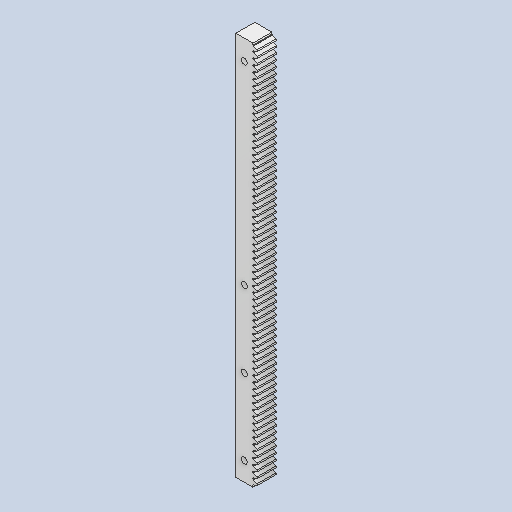
# Autodesk Inventor part: ラックM1‗8
Saved by Autodesk Inventor 2023 (Build 270158000, 158)
## iProperties
Created: 2022-09-12
Part Number: ラックM1‗8
Material: PC/ABS プラスチック
Document SubType Name: Modeling
Designer: 野口　裕太
Density: 0.357273 g/cm^3
Appearance: 滑らか - 白
Author: 野口　裕太
Autodesk Inventor part; units mm, degrees
(part 1 of 4)
ref_plane "YZ Plane" through (0, 0, 0) normal (1, 0, 0) x (0, 1, 0)
ref_plane "XZ Plane" through (0, 0, 0) normal (0, 1, 0) x (-1, 0, 0)
ref_plane "XY Plane" through (0, 0, 0) normal (0, 0, 1) x (1, 0, 0)
sketch "スケッチ1" plane through (0, 0, 0) normal (0, 0, 1) x (1, 0, 0)
  line L0 (8.75, 0) -> (8.75, 0.1735)
  line L1 (8.75, 0.1735) -> (8.7511, 0.1906)
  line L2 (8.7511, 0.1906) -> (8.7542, 0.2077)
  line L3 (8.7542, 0.2077) -> (8.7595, 0.2248)
  line L4 (8.7595, 0.2248) -> (8.7669, 0.2417)
  line L5 (8.7669, 0.2417) -> (8.7764, 0.2586)
  line L6 (8.7764, 0.2586) -> (8.788, 0.2753)
  line L7 (8.788, 0.2753) -> (8.8018, 0.2918)
  line L8 (8.8018, 0.2918) -> (8.8176, 0.3081)
  line L9 (8.8176, 0.3081) -> (8.8355, 0.3242)
  line L10 (8.8355, 0.3242) -> (8.8556, 0.34)
  line L11 (8.8556, 0.34) -> (8.8777, 0.3556)
  line L12 (8.8777, 0.3556) -> (8.9019, 0.3708)
  line L13 (8.9019, 0.3708) -> (8.9282, 0.3857)
  line L14 (8.9282, 0.3857) -> (8.9566, 0.4002)
  line L15 (8.9566, 0.4002) -> (8.9871, 0.4143)
  line L16 (8.9871, 0.4143) -> (9.0196, 0.428)
  line L17 (9.0196, 0.428) -> (9.0542, 0.4412)
  line L18 (9.0542, 0.4412) -> (11, 1.1494)
  line L19 (11, 1.1494) -> (11, 1.5708)
  line L20 (8.788, 2.8663) -> (8.8018, 2.8498)
  line L21 (8.8018, 2.8498) -> (8.8176, 2.8335)
  line L22 (8.8176, 2.8335) -> (8.8355, 2.8174)
  line L23 (8.8355, 2.8174) -> (8.8556, 2.8016)
  line L24 (8.8556, 2.8016) -> (8.8777, 2.786)
  line L25 (8.9019, 2.7708) -> (8.9282, 2.7559)
  line L26 (8.9282, 2.7559) -> (8.9566, 2.7414)
  line L27 (8.9566, 2.7414) -> (8.9871, 2.7273)
  line L28 (8.9871, 2.7273) -> (9.0196, 2.7136)
  line L29 (9.0196, 2.7136) -> (9.0542, 2.7004)
  line L30 (9.0542, 2.7004) -> (11, 1.9922)
  line L31 (11, 1.9922) -> (11, 1.5708)
  line L32 (8.75, 3.1416) -> (8.75, 2.9681)
  line L33 (8.75, 2.9681) -> (8.7511, 2.951)
  line L34 (8.7511, 2.951) -> (8.7542, 2.9339)
  line L35 (8.7764, 2.883) -> (8.788, 2.8663)
  line L36 (8.7669, 2.8999) -> (8.7764, 2.883)
  line L37 (8.7595, 2.9168) -> (8.7669, 2.8999)
  line L38 (8.7542, 2.9339) -> (8.7595, 2.9168)
  line L39 (8.8777, 2.786) -> (8.9019, 2.7708)
  line L40 (8.75, 3.1416) -> (7.1265, 3.1416)
  line L41 (8.8777, 5.9276) -> (8.9019, 5.9124)
  line L42 (8.9019, 5.9124) -> (8.9282, 5.8975)
  line L43 (8.9282, 5.8975) -> (8.9566, 5.883)
  line L44 (8.9566, 5.883) -> (8.9871, 5.8689)
  line L45 (8.9871, 5.8689) -> (9.0196, 5.8552)
  line L46 (9.0196, 5.8552) -> (9.0542, 5.842)
  line L47 (9.0542, 5.842) -> (11, 5.1338)
  line L48 (11, 5.1338) -> (11, 4.7124)
  line L49 (9.0542, 3.5828) -> (11, 4.291)
  line L50 (8.75, 6.2832) -> (8.75, 6.1097)
  line L51 (8.75, 6.1097) -> (8.7511, 6.0926)
  line L52 (8.7511, 6.0926) -> (8.7542, 6.0755)
  line L53 (8.7542, 6.0755) -> (8.7595, 6.0584)
  line L54 (8.8556, 5.9431) -> (8.8777, 5.9276)
  line L55 (8.8355, 5.959) -> (8.8556, 5.9431)
  line L56 (8.8176, 5.9751) -> (8.8355, 5.959)
  line L57 (8.8018, 5.9914) -> (8.8176, 5.9751)
  line L58 (8.788, 6.0079) -> (8.8018, 5.9914)
  line L59 (8.7764, 6.0246) -> (8.788, 6.0079)
  line L60 (8.7669, 6.0415) -> (8.7764, 6.0246)
  line L61 (8.7595, 6.0584) -> (8.7669, 6.0415)
  line L62 (8.9871, 3.5559) -> (9.0196, 3.5695)
  line L63 (8.9566, 3.5418) -> (8.9871, 3.5559)
  line L64 (8.9282, 3.5273) -> (8.9566, 3.5418)
  line L65 (8.9019, 3.5124) -> (8.9282, 3.5273)
  line L66 (8.8777, 3.4972) -> (8.9019, 3.5124)
  line L67 (8.8556, 3.4816) -> (8.8777, 3.4972)
  line L68 (8.8355, 3.4658) -> (8.8556, 3.4816)
  line L69 (8.8176, 3.4497) -> (8.8355, 3.4658)
  line L70 (8.8018, 3.4334) -> (8.8176, 3.4497)
  line L71 (11, 4.291) -> (11, 4.7124)
  line L72 (9.0196, 3.5695) -> (9.0542, 3.5828)
  line L73 (8.788, 3.4169) -> (8.8018, 3.4334)
  line L74 (8.7764, 3.4002) -> (8.788, 3.4169)
  line L75 (8.7595, 3.3664) -> (8.7669, 3.3833)
  line L76 (8.7542, 3.3493) -> (8.7595, 3.3664)
  line L77 (8.7511, 3.3322) -> (8.7542, 3.3493)
  line L78 (8.75, 3.3151) -> (8.7511, 3.3322)
  line L79 (8.75, 3.1416) -> (8.75, 3.3151)
  line L80 (8.7669, 3.3833) -> (8.7764, 3.4002)
  line L81 (8.75, 6.2832) -> (7.8414, 6.2832)
  line L82 (8.9282, 12.1807) -> (8.9566, 12.1662)
  line L83 (8.9566, 12.1662) -> (8.9871, 12.1521)
  line L84 (8.9871, 12.1521) -> (9.0196, 12.1384)
  line L85 (9.0196, 12.1384) -> (9.0542, 12.1252)
  line L86 (9.0542, 12.1252) -> (11, 11.417)
  line L87 (11, 11.417) -> (11, 10.9956)
  line L88 (11, 10.5741) -> (11, 10.9956)
  line L89 (9.0542, 9.8659) -> (11, 10.5741)
  line L90 (9.0196, 9.8527) -> (9.0542, 9.8659)
  line L91 (8.9871, 9.8391) -> (9.0196, 9.8527)
  line L92 (8.9566, 9.825) -> (8.9871, 9.8391)
  line L93 (8.9282, 9.8105) -> (8.9566, 9.825)
  line L94 (8.9019, 9.7956) -> (8.9282, 9.8105)
  line L95 (8.8777, 9.7804) -> (8.9019, 9.7956)
  line L96 (8.788, 9.7001) -> (8.8018, 9.7166)
  line L97 (8.8018, 9.7166) -> (8.8176, 9.7329)
  line L98 (8.8556, 9.7648) -> (8.8777, 9.7804)
  line L99 (8.8355, 9.749) -> (8.8556, 9.7648)
  line L100 (8.8176, 9.7329) -> (8.8355, 9.749)
  line L101 (8.7764, 9.6834) -> (8.788, 9.7001)
  line L102 (8.7669, 9.6665) -> (8.7764, 9.6834)
  line L103 (8.7595, 9.6495) -> (8.7669, 9.6665)
  line L104 (8.7542, 9.6325) -> (8.7595, 9.6495)
  line L105 (8.7511, 9.6154) -> (8.7542, 9.6325)
  line L106 (8.75, 9.5983) -> (8.7511, 9.6154)
  line L107 (8.75, 9.4248) -> (8.75, 9.5983)
  line L108 (8.75, 9.4248) -> (8.75, 9.2513)
  line L109 (8.75, 9.2513) -> (8.7511, 9.2342)
  line L110 (8.7511, 9.2342) -> (8.7542, 9.2171)
  line L111 (8.7542, 9.2171) -> (8.7595, 9.2)
  line L112 (8.7595, 9.2) -> (8.7669, 9.183)
  line L113 (8.7669, 9.183) -> (8.7764, 9.1662)
  line L114 (8.7764, 9.1662) -> (8.788, 9.1495)
  line L115 (8.8018, 9.133) -> (8.8176, 9.1167)
  line L116 (8.8176, 9.1167) -> (8.8355, 9.1006)
  line L117 (8.8355, 9.1006) -> (8.8556, 9.0847)
  line L118 (8.8556, 9.0847) -> (8.8777, 9.0692)
  line L119 (8.8777, 9.0692) -> (8.9019, 9.054)
  line L120 (8.9019, 9.054) -> (8.9282, 9.0391)
  line L121 (8.788, 9.1495) -> (8.8018, 9.133)
  line L122 (8.75, 12.5664) -> (8.75, 12.3929)
  line L123 (8.75, 12.3929) -> (8.7511, 12.3758)
  line L124 (8.7511, 12.3758) -> (8.7542, 12.3586)
  line L125 (8.7542, 12.3586) -> (8.7595, 12.3416)
  line L126 (8.9019, 12.1956) -> (8.9282, 12.1807)
  line L127 (8.8777, 12.2108) -> (8.9019, 12.1956)
  line L128 (8.8556, 12.2263) -> (8.8777, 12.2108)
  line L129 (8.8355, 12.2422) -> (8.8556, 12.2263)
  line L130 (8.8176, 12.2583) -> (8.8355, 12.2422)
  line L131 (8.8018, 12.2746) -> (8.8176, 12.2583)
  line L132 (8.788, 12.2911) -> (8.8018, 12.2746)
  line L133 (8.7764, 12.3078) -> (8.788, 12.2911)
  line L134 (8.7669, 12.3246) -> (8.7764, 12.3078)
  line L135 (8.7595, 12.3416) -> (8.7669, 12.3246)
  line L136 (8.8777, 6.6388) -> (8.9019, 6.654)
  line L137 (8.9019, 6.654) -> (8.9282, 6.6689)
  line L138 (8.75, 6.2832) -> (8.75, 6.4567)
  line L139 (8.75, 6.4567) -> (8.7511, 6.4738)
  line L140 (8.7511, 6.4738) -> (8.7542, 6.4909)
  line L141 (8.7542, 6.4909) -> (8.7595, 6.508)
  line L142 (8.8556, 6.6232) -> (8.8777, 6.6388)
  line L143 (8.8355, 6.6074) -> (8.8556, 6.6232)
  line L144 (8.8176, 6.5913) -> (8.8355, 6.6074)
  line L145 (8.8018, 6.575) -> (8.8176, 6.5913)
  line L146 (8.788, 6.5585) -> (8.8018, 6.575)
  line L147 (8.7764, 6.5418) -> (8.788, 6.5585)
  line L148 (8.7669, 6.5249) -> (8.7764, 6.5418)
  line L149 (8.7595, 6.508) -> (8.7669, 6.5249)
  line L150 (8.9282, 6.6689) -> (8.9566, 6.6834)
  line L151 (8.9566, 6.6834) -> (8.9871, 6.6975)
  line L152 (8.9871, 6.6975) -> (9.0196, 6.7111)
  line L153 (9.0196, 6.7111) -> (9.0542, 6.7243)
  line L154 (9.0542, 6.7243) -> (11, 7.4326)
  line L155 (11, 7.4326) -> (11, 7.854)
  line L156 (9.0542, 8.9836) -> (11, 8.2754)
  line L157 (8.9871, 9.0105) -> (9.0196, 8.9968)
  line L158 (8.9566, 9.0246) -> (8.9871, 9.0105)
  line L159 (9.0196, 8.9968) -> (9.0542, 8.9836)
  line L160 (11, 8.2754) -> (11, 7.854)
  line L161 (8.9282, 9.0391) -> (8.9566, 9.0246)
  line L162 (8.75, 12.5664) -> (7.1265, 12.5664)
  line L163 (8.9871, 24.7185) -> (9.0196, 24.7048)
  line L164 (9.0196, 24.7048) -> (9.0542, 24.6916)
  line L165 (9.0542, 24.6916) -> (11, 23.9834)
  line L166 (11, 23.9834) -> (11, 23.5619)
  line L167 (8.75, 25.1327) -> (8.75, 24.9593)
  line L168 (8.75, 24.9593) -> (8.7511, 24.9421)
  line L169 (8.7511, 24.9421) -> (8.7542, 24.925)
  line L170 (8.7542, 24.925) -> (8.7595, 24.908)
  line L171 (8.8176, 24.8246) -> (8.8355, 24.8085)
  line L172 (8.8355, 24.8085) -> (8.8556, 24.7927)
  line L173 (8.9282, 24.7471) -> (8.9566, 24.7326)
  line L174 (8.9019, 24.7619) -> (8.9282, 24.7471)
  line L175 (8.8777, 24.7772) -> (8.9019, 24.7619)
  line L176 (8.8556, 24.7927) -> (8.8777, 24.7772)
  line L177 (8.8018, 24.8409) -> (8.8176, 24.8246)
  line L178 (8.788, 24.8575) -> (8.8018, 24.8409)
  line L179 (8.7764, 24.8742) -> (8.788, 24.8575)
  line L180 (8.7669, 24.891) -> (8.7764, 24.8742)
  line L181 (8.7595, 24.908) -> (8.7669, 24.891)
  line L182 (8.9566, 24.7326) -> (8.9871, 24.7185)
  line L183 (11, 23.1405) -> (11, 23.5619)
  line L184 (9.0542, 22.4323) -> (11, 23.1405)
  line L185 (9.0196, 22.4191) -> (9.0542, 22.4323)
  line L186 (8.9871, 22.4054) -> (9.0196, 22.4191)
  line L187 (8.9566, 22.3913) -> (8.9871, 22.4054)
  line L188 (8.9282, 22.3768) -> (8.9566, 22.3913)
  line L189 (8.9019, 22.362) -> (8.9282, 22.3768)
  line L190 (8.788, 22.2664) -> (8.8018, 22.2829)
  line L191 (8.8018, 22.2829) -> (8.8176, 22.2993)
  line L192 (8.8176, 22.2993) -> (8.8355, 22.3154)
  line L193 (8.8777, 22.3467) -> (8.9019, 22.362)
  line L194 (8.8556, 22.3312) -> (8.8777, 22.3467)
  line L195 (8.8355, 22.3154) -> (8.8556, 22.3312)
  line L196 (8.7764, 22.2497) -> (8.788, 22.2664)
  line L197 (8.7669, 22.2329) -> (8.7764, 22.2497)
  line L198 (8.7595, 22.2159) -> (8.7669, 22.2329)
  line L199 (8.7542, 22.1989) -> (8.7595, 22.2159)
  line L200 (8.7511, 22.1818) -> (8.7542, 22.1989)
  line L201 (8.75, 22.1646) -> (8.7511, 22.1818)
  line L202 (8.75, 21.9911) -> (8.75, 22.1646)
  line L203 (8.7764, 21.7326) -> (8.788, 21.7159)
  line L204 (8.788, 21.7159) -> (8.8018, 21.6994)
  line L205 (8.8018, 21.6994) -> (8.8176, 21.683)
  line L206 (8.8355, 21.6669) -> (8.8556, 21.6511)
  line L207 (8.8556, 21.6511) -> (8.8777, 21.6356)
  line L208 (8.8777, 21.6356) -> (8.9019, 21.6203)
  line L209 (8.9019, 21.6203) -> (8.9282, 21.6055)
  line L210 (8.9282, 21.6055) -> (8.9566, 21.591)
  line L211 (8.8176, 21.683) -> (8.8355, 21.6669)
  line L212 (8.8777, 19.2051) -> (8.9019, 19.2204)
  line L213 (8.9019, 19.2204) -> (8.9282, 19.2352)
  line L214 (8.75, 18.8496) -> (8.75, 19.023)
  line L215 (8.75, 19.023) -> (8.7511, 19.0402)
  line L216 (8.7511, 19.0402) -> (8.7542, 19.0573)
  line L217 (8.7542, 19.0573) -> (8.7595, 19.0743)
  line L218 (8.8556, 19.1896) -> (8.8777, 19.2051)
  line L219 (8.8355, 19.1738) -> (8.8556, 19.1896)
  line L220 (8.8176, 19.1577) -> (8.8355, 19.1738)
  line L221 (8.8018, 19.1414) -> (8.8176, 19.1577)
  line L222 (8.7595, 19.0743) -> (8.7669, 19.0913)
  line L223 (8.7669, 19.0913) -> (8.7764, 19.1081)
  line L224 (8.788, 19.1248) -> (8.8018, 19.1414)
  line L225 (8.7764, 19.1081) -> (8.788, 19.1248)
  line L226 (8.9282, 19.2352) -> (8.9566, 19.2497)
  line L227 (8.9566, 19.2497) -> (8.9871, 19.2638)
  line L228 (8.9871, 19.2638) -> (9.0196, 19.2775)
  line L229 (9.0196, 19.2775) -> (9.0542, 19.2907)
  line L230 (9.0542, 19.2907) -> (11, 19.9989)
  line L231 (11, 19.9989) -> (11, 20.4204)
  line L232 (9.0542, 21.55) -> (11, 20.8418)
  line L233 (8.9871, 21.5769) -> (9.0196, 21.5632)
  line L234 (9.0196, 21.5632) -> (9.0542, 21.55)
  line L235 (11, 20.8418) -> (11, 20.4204)
  line L236 (8.9566, 21.591) -> (8.9871, 21.5769)
  line L237 (8.7669, 21.7494) -> (8.7764, 21.7326)
  line L238 (8.7595, 21.7664) -> (8.7669, 21.7494)
  line L239 (8.7542, 21.7834) -> (8.7595, 21.7664)
  line L240 (8.7511, 21.8005) -> (8.7542, 21.7834)
  line L241 (8.75, 21.8177) -> (8.7511, 21.8005)
  line L242 (8.75, 21.9911) -> (8.75, 21.8177)
  line L243 (8.9566, 12.9666) -> (8.9871, 12.9807)
  line L244 (8.9871, 12.9807) -> (9.0196, 12.9943)
  line L245 (9.0196, 12.9943) -> (9.0542, 13.0075)
  line L246 (9.0542, 15.2668) -> (11, 14.5586)
  line L247 (9.0542, 13.0075) -> (11, 13.7157)
  line L248 (11, 14.5586) -> (11, 14.1372)
  line L249 (11, 13.7157) -> (11, 14.1372)
  line L250 (8.7542, 15.5002) -> (8.7595, 15.4832)
  line L251 (8.7511, 15.5173) -> (8.7542, 15.5002)
  line L252 (8.75, 15.5345) -> (8.7511, 15.5173)
  line L253 (8.75, 15.708) -> (8.75, 15.5345)
  line L254 (8.75, 15.708) -> (8.75, 15.8814)
  line L255 (8.7595, 15.4832) -> (8.7669, 15.4662)
  line L256 (9.0196, 15.28) -> (9.0542, 15.2668)
  line L257 (8.9871, 15.2937) -> (9.0196, 15.28)
  line L258 (8.9566, 15.3078) -> (8.9871, 15.2937)
  line L259 (8.9282, 15.3223) -> (8.9566, 15.3078)
  line L260 (8.9019, 15.3372) -> (8.9282, 15.3223)
  line L261 (8.8777, 15.3524) -> (8.9019, 15.3372)
  line L262 (8.8556, 15.3679) -> (8.8777, 15.3524)
  line L263 (8.8355, 15.3838) -> (8.8556, 15.3679)
  line L264 (8.8176, 15.3998) -> (8.8355, 15.3838)
  line L265 (8.8018, 15.4162) -> (8.8176, 15.3998)
  line L266 (8.788, 15.4327) -> (8.8018, 15.4162)
  line L267 (8.7764, 15.4494) -> (8.788, 15.4327)
  line L268 (8.7669, 15.4662) -> (8.7764, 15.4494)
  line L269 (8.8556, 16.048) -> (8.8777, 16.0635)
  line L270 (8.8777, 16.0635) -> (8.9019, 16.0788)
  line L271 (8.9019, 16.0788) -> (8.9282, 16.0936)
  line L272 (8.9282, 16.0936) -> (8.9566, 16.1082)
  line L273 (8.9566, 16.1082) -> (8.9871, 16.1222)
  line L274 (8.9871, 16.1222) -> (9.0196, 16.1359)
  line L275 (8.75, 15.8814) -> (8.7511, 15.8986)
  line L276 (8.7511, 15.8986) -> (8.7542, 15.9157)
  line L277 (8.7542, 15.9157) -> (8.7595, 15.9327)
  line L278 (8.7595, 15.9327) -> (8.7669, 15.9497)
  line L279 (8.7669, 15.9497) -> (8.7764, 15.9665)
  line L280 (8.7764, 15.9665) -> (8.788, 15.9832)
  line L281 (8.788, 15.9832) -> (8.8018, 15.9998)
  line L282 (8.8018, 15.9998) -> (8.8176, 16.0161)
  line L283 (8.8176, 16.0161) -> (8.8355, 16.0322)
  line L284 (8.8355, 16.0322) -> (8.8556, 16.048)
  line L285 (8.75, 18.8496) -> (8.75, 18.6761)
  line L286 (8.75, 18.6761) -> (8.7511, 18.6589)
  line L287 (8.7511, 18.6589) -> (8.7542, 18.6418)
  line L288 (8.7542, 18.6418) -> (8.7595, 18.6248)
  line L289 (8.7595, 18.6248) -> (8.7669, 18.6078)
  line L290 (8.7764, 18.591) -> (8.788, 18.5743)
  line L291 (8.788, 18.5743) -> (8.8018, 18.5578)
  line L292 (8.8018, 18.5578) -> (8.8176, 18.5414)
  line L293 (8.8176, 18.5414) -> (8.8355, 18.5253)
  line L294 (8.8355, 18.5253) -> (8.8556, 18.5095)
  line L295 (8.8556, 18.5095) -> (8.8777, 18.494)
  line L296 (8.7669, 18.6078) -> (8.7764, 18.591)
  line L297 (8.8777, 18.494) -> (8.9019, 18.4787)
  line L298 (8.9019, 18.4787) -> (8.9282, 18.4639)
  line L299 (8.9282, 18.4639) -> (8.9566, 18.4494)
  line L300 (8.9566, 18.4494) -> (8.9871, 18.4353)
  line L301 (8.9871, 18.4353) -> (9.0196, 18.4216)
  line L302 (9.0196, 18.4216) -> (9.0542, 18.4084)
  line L303 (8.9282, 12.9521) -> (8.9566, 12.9666)
  line L304 (8.9019, 12.9372) -> (8.9282, 12.9521)
  line L305 (8.8777, 12.922) -> (8.9019, 12.9372)
  line L306 (8.8355, 12.8906) -> (8.8556, 12.9064)
  line L307 (8.8176, 12.8745) -> (8.8355, 12.8906)
  line L308 (8.8018, 12.8582) -> (8.8176, 12.8745)
  line L309 (8.788, 12.8416) -> (8.8018, 12.8582)
  line L310 (8.7764, 12.8249) -> (8.788, 12.8416)
  line L311 (8.7669, 12.8081) -> (8.7764, 12.8249)
  line L312 (8.7595, 12.7911) -> (8.7669, 12.8081)
  line L313 (8.7542, 12.7741) -> (8.7595, 12.7911)
  line L314 (8.7511, 12.757) -> (8.7542, 12.7741)
  line L315 (8.75, 12.7399) -> (8.7511, 12.757)
  line L316 (8.75, 12.5664) -> (8.75, 12.7399)
  line L317 (8.8556, 12.9064) -> (8.8777, 12.922)
  line L318 (9.0542, 18.4084) -> (11, 17.7002)
  line L319 (11, 17.7002) -> (11, 17.2788)
  line L320 (9.0196, 16.1359) -> (9.0542, 16.1491)
  line L321 (11, 16.8573) -> (11, 17.2788)
  line L322 (9.0542, 16.1491) -> (11, 16.8573)
  line L323 (8.75, 25.1327) -> (7.9383, 25.1327)
  line L324 (8.75, 50.2655) -> (8.75, 50.092)
  line L325 (8.75, 50.092) -> (8.7511, 50.0749)
  line L326 (8.7511, 50.0749) -> (8.7542, 50.0578)
  line L327 (8.7542, 50.0578) -> (8.7595, 50.0407)
  line L328 (8.7595, 50.0407) -> (8.7669, 50.0238)
  line L329 (8.7669, 50.0238) -> (8.7764, 50.0069)
  line L330 (8.9019, 49.8947) -> (8.9282, 49.8798)
  line L331 (8.9282, 49.8798) -> (8.9566, 49.8653)
  line L332 (8.7764, 50.0069) -> (8.788, 49.9902)
  line L333 (8.9566, 49.8653) -> (8.9871, 49.8512)
  line L334 (8.788, 47.3992) -> (8.8018, 47.4157)
  line L335 (8.8018, 47.4157) -> (8.8176, 47.432)
  line L336 (8.7764, 47.3825) -> (8.788, 47.3992)
  line L337 (8.7669, 47.3656) -> (8.7764, 47.3825)
  line L338 (8.7595, 47.3487) -> (8.7669, 47.3656)
  line L339 (8.7542, 47.3316) -> (8.7595, 47.3487)
  line L340 (8.7511, 47.3145) -> (8.7542, 47.3316)
  line L341 (8.75, 47.2974) -> (8.7511, 47.3145)
  line L342 (8.75, 47.1239) -> (8.75, 47.2974)
  line L343 (8.8176, 47.432) -> (8.8355, 47.4481)
  line L344 (8.9871, 49.8512) -> (9.0196, 49.8375)
  line L345 (9.0196, 49.8375) -> (9.0542, 49.8243)
  line L346 (8.8777, 49.9099) -> (8.9019, 49.8947)
  line L347 (8.8556, 49.9254) -> (8.8777, 49.9099)
  line L348 (8.8355, 49.9413) -> (8.8556, 49.9254)
  line L349 (8.8176, 49.9574) -> (8.8355, 49.9413)
  line L350 (8.8018, 49.9737) -> (8.8176, 49.9574)
  line L351 (9.0542, 49.8243) -> (11, 49.1161)
  line L352 (9.0542, 47.5651) -> (11, 48.2733)
  line L353 (11, 48.2733) -> (11, 48.6947)
  line L354 (11, 49.1161) -> (11, 48.6947)
  line L355 (8.788, 49.9902) -> (8.8018, 49.9737)
  line L356 (8.75, 47.1239) -> (8.75, 46.9504)
  line L357 (8.75, 46.9504) -> (8.7511, 46.9333)
  line L358 (8.7511, 46.9333) -> (8.7542, 46.9162)
  line L359 (8.7542, 46.9162) -> (8.7595, 46.8991)
  line L360 (8.7595, 46.8991) -> (8.7669, 46.8822)
  line L361 (8.7669, 46.8822) -> (8.7764, 46.8653)
  line L362 (8.7764, 46.8653) -> (8.788, 46.8486)
  line L363 (8.788, 46.8486) -> (8.8018, 46.8321)
  line L364 (8.8018, 46.8321) -> (8.8176, 46.8158)
  line L365 (8.8777, 44.3379) -> (8.9019, 44.3531)
  line L366 (8.9019, 44.3531) -> (8.9282, 44.368)
  line L367 (8.9282, 44.368) -> (8.9566, 44.3825)
  line L368 (8.9566, 44.3825) -> (8.9871, 44.3966)
  line L369 (8.7595, 44.2071) -> (8.7669, 44.224)
  line L370 (8.7669, 44.224) -> (8.7764, 44.2409)
  line L371 (8.7764, 44.2409) -> (8.788, 44.2576)
  line L372 (8.788, 44.2576) -> (8.8018, 44.2741)
  line L373 (8.8018, 44.2741) -> (8.8176, 44.2904)
  line L374 (8.8176, 44.2904) -> (8.8355, 44.3065)
  line L375 (8.8556, 44.3223) -> (8.8777, 44.3379)
  line L376 (8.8355, 44.3065) -> (8.8556, 44.3223)
  line L377 (8.9871, 44.3966) -> (9.0196, 44.4103)
  line L378 (9.0196, 44.4103) -> (9.0542, 44.4235)
  line L379 (9.0542, 44.4235) -> (11, 45.1317)
  line L380 (11, 45.1317) -> (11, 45.5531)
  line L381 (9.0542, 46.6827) -> (11, 45.9745)
  line L382 (8.9871, 46.7096) -> (9.0196, 46.6959)
  line L383 (8.8355, 46.7997) -> (8.8556, 46.7838)
  line L384 (8.8556, 46.7838) -> (8.8777, 46.7683)
  line L385 (8.8777, 46.7683) -> (8.9019, 46.7531)
  line L386 (8.9019, 46.7531) -> (8.9282, 46.7382)
  line L387 (8.9282, 46.7382) -> (8.9566, 46.7237)
  line L388 (8.9566, 46.7237) -> (8.9871, 46.7096)
  line L389 (9.0196, 46.6959) -> (9.0542, 46.6827)
  line L390 (11, 45.9745) -> (11, 45.5531)
  line L391 (8.8176, 46.8158) -> (8.8355, 46.7997)
  line L392 (8.8355, 47.4481) -> (8.8556, 47.4639)
  line L393 (8.8556, 47.4639) -> (8.8777, 47.4795)
  line L394 (8.8777, 47.4795) -> (8.9019, 47.4947)
  line L395 (8.9019, 47.4947) -> (8.9282, 47.5096)
  line L396 (8.9282, 47.5096) -> (8.9566, 47.5241)
  line L397 (8.9566, 47.5241) -> (8.9871, 47.5382)
  line L398 (8.9871, 47.5382) -> (9.0196, 47.5518)
  line L399 (9.0196, 47.5518) -> (9.0542, 47.5651)
  line L400 (8.7764, 40.5821) -> (8.788, 40.5654)
  line L401 (8.7669, 40.599) -> (8.7764, 40.5821)
  line L402 (8.7595, 40.6159) -> (8.7669, 40.599)
  line L403 (8.7542, 40.633) -> (8.7595, 40.6159)
  line L404 (8.7511, 40.6501) -> (8.7542, 40.633)
  line L405 (8.75, 40.6672) -> (8.7511, 40.6501)
  line L406 (8.75, 40.8407) -> (8.75, 40.6672)
  line L407 (8.788, 40.5654) -> (8.8018, 40.5489)
  line L408 (8.9871, 38.1134) -> (9.0196, 38.1271)
  line L409 (9.0196, 38.1271) -> (9.0542, 38.1403)
  line L410 (9.0542, 38.1403) -> (11, 38.8485)
  line L411 (11, 38.8485) -> (11, 39.2699)
  line L412 (11, 39.6913) -> (11, 39.2699)
  line L413 (9.0542, 40.3995) -> (11, 39.6913)
  line L414 (9.0196, 40.4128) -> (9.0542, 40.3995)
  line L415 (8.8018, 40.5489) -> (8.8176, 40.5326)
  line L416 (8.8355, 40.5165) -> (8.8556, 40.5007)
  line L417 (8.8556, 40.5007) -> (8.8777, 40.4851)
  line L418 (8.8777, 40.4851) -> (8.9019, 40.4699)
  line L419 (8.9019, 40.4699) -> (8.9282, 40.455)
  line L420 (8.9282, 40.455) -> (8.9566, 40.4405)
  line L421 (8.9566, 40.4405) -> (8.9871, 40.4264)
  line L422 (8.9871, 40.4264) -> (9.0196, 40.4128)
  line L423 (8.8176, 40.5326) -> (8.8355, 40.5165)
  line L424 (8.75, 40.8407) -> (8.75, 41.0142)
  line L425 (8.75, 41.0142) -> (8.7511, 41.0313)
  line L426 (8.7542, 41.0484) -> (8.7595, 41.0655)
  line L427 (8.7595, 41.0655) -> (8.7669, 41.0824)
  line L428 (8.7669, 41.0824) -> (8.7764, 41.0993)
  line L429 (8.7764, 41.0993) -> (8.788, 41.116)
  line L430 (8.7511, 41.0313) -> (8.7542, 41.0484)
  line L431 (8.788, 41.116) -> (8.8018, 41.1325)
  line L432 (8.8176, 41.1488) -> (8.8355, 41.1649)
  line L433 (8.8355, 41.1649) -> (8.8556, 41.1807)
  line L434 (8.8556, 41.1807) -> (8.8777, 41.1963)
  line L435 (8.8777, 41.1963) -> (8.9019, 41.2115)
  line L436 (8.9019, 41.2115) -> (8.9282, 41.2264)
  line L437 (8.9282, 41.2264) -> (8.9566, 41.2409)
  line L438 (8.9566, 41.2409) -> (8.9871, 41.255)
  line L439 (8.8018, 41.1325) -> (8.8176, 41.1488)
  line L440 (8.9282, 38.0848) -> (8.9566, 38.0993)
  line L441 (8.9566, 38.0993) -> (8.9871, 38.1134)
  line L442 (8.75, 37.6991) -> (8.75, 37.8726)
  line L443 (8.75, 37.8726) -> (8.7511, 37.8897)
  line L444 (8.7511, 37.8897) -> (8.7542, 37.9068)
  line L445 (8.7542, 37.9068) -> (8.7595, 37.9239)
  line L446 (8.9019, 38.0699) -> (8.9282, 38.0848)
  line L447 (8.8777, 38.0547) -> (8.9019, 38.0699)
  line L448 (8.8556, 38.0392) -> (8.8777, 38.0547)
  line L449 (8.8355, 38.0233) -> (8.8556, 38.0392)
  line L450 (8.7595, 37.9239) -> (8.7669, 37.9408)
  line L451 (8.7764, 37.9577) -> (8.788, 37.9744)
  line L452 (8.788, 37.9744) -> (8.8018, 37.9909)
  line L453 (8.8018, 37.9909) -> (8.8176, 38.0072)
  line L454 (8.8176, 38.0072) -> (8.8355, 38.0233)
  line L455 (8.7669, 37.9408) -> (8.7764, 37.9577)
  line L456 (8.75, 43.9823) -> (8.75, 44.1558)
  line L457 (8.75, 44.1558) -> (8.7511, 44.1729)
  line L458 (8.7511, 44.1729) -> (8.7542, 44.19)
  line L459 (8.75, 43.9823) -> (8.75, 43.8088)
  line L460 (8.75, 43.8088) -> (8.7511, 43.7917)
  line L461 (8.7511, 43.7917) -> (8.7542, 43.7746)
  line L462 (8.7542, 43.7746) -> (8.7595, 43.7575)
  line L463 (8.7595, 43.7575) -> (8.7669, 43.7406)
  line L464 (8.7669, 43.7406) -> (8.7764, 43.7237)
  line L465 (8.7764, 43.7237) -> (8.788, 43.707)
  line L466 (8.788, 43.707) -> (8.8018, 43.6905)
  line L467 (8.8018, 43.6905) -> (8.8176, 43.6742)
  line L468 (8.7542, 44.19) -> (8.7595, 44.2071)
  line L469 (8.8777, 43.6267) -> (8.9019, 43.6115)
  line L470 (8.8176, 43.6742) -> (8.8355, 43.6581)
  line L471 (8.8355, 43.6581) -> (8.8556, 43.6423)
  line L472 (8.8556, 43.6423) -> (8.8777, 43.6267)
  line L473 (8.9019, 43.6115) -> (8.9282, 43.5966)
  line L474 (8.9282, 43.5966) -> (8.9566, 43.5821)
  line L475 (8.9566, 43.5821) -> (8.9871, 43.568)
  line L476 (8.9871, 43.568) -> (9.0196, 43.5543)
  line L477 (9.0196, 43.5543) -> (9.0542, 43.5411)
  line L478 (9.0196, 41.2687) -> (9.0542, 41.2819)
  line L479 (9.0542, 41.2819) -> (11, 41.9901)
  line L480 (11, 41.9901) -> (11, 42.4115)
  line L481 (11, 42.8329) -> (11, 42.4115)
  line L482 (9.0542, 43.5411) -> (11, 42.8329)
  line L483 (8.9871, 41.255) -> (9.0196, 41.2687)
  line L484 (8.75, 25.3062) -> (8.7511, 25.3234)
  line L485 (8.75, 25.1327) -> (8.75, 25.3062)
  line L486 (9.0542, 25.5739) -> (11, 26.2821)
  line L487 (11, 26.2821) -> (11, 26.7035)
  line L488 (11, 27.125) -> (11, 26.7035)
  line L489 (9.0542, 27.8332) -> (11, 27.125)
  line L490 (9.0196, 27.8464) -> (9.0542, 27.8332)
  line L491 (8.9871, 27.86) -> (9.0196, 27.8464)
  line L492 (8.7764, 28.0158) -> (8.788, 27.9991)
  line L493 (8.788, 27.9991) -> (8.8018, 27.9825)
  line L494 (8.8018, 27.9825) -> (8.8176, 27.9662)
  line L495 (8.8176, 27.9662) -> (8.8355, 27.9501)
  line L496 (8.8355, 27.9501) -> (8.8556, 27.9343)
  line L497 (8.8556, 27.9343) -> (8.8777, 27.9188)
  line L498 (8.8777, 27.9188) -> (8.9019, 27.9035)
  line L499 (8.9019, 27.9035) -> (8.9282, 27.8886)
  line L500 (8.9282, 27.8886) -> (8.9566, 27.8741)
  line L501 (8.9566, 27.8741) -> (8.9871, 27.86)
  line L502 (8.7669, 28.0326) -> (8.7764, 28.0158)
  line L503 (8.7595, 28.0496) -> (8.7669, 28.0326)
  line L504 (8.7542, 28.0666) -> (8.7595, 28.0496)
  line L505 (8.7511, 28.0837) -> (8.7542, 28.0666)
  line L506 (8.75, 28.1008) -> (8.7511, 28.0837)
  line L507 (8.75, 28.2743) -> (8.75, 28.1008)
  line L508 (8.75, 28.2743) -> (8.75, 28.4478)
  line L509 (8.75, 28.4478) -> (8.7511, 28.465)
  line L510 (8.7511, 28.465) -> (8.7542, 28.4821)
  line L511 (8.7542, 28.4821) -> (8.7595, 28.4991)
  line L512 (8.7595, 28.4991) -> (8.7669, 28.5161)
  line L513 (8.7669, 28.5161) -> (8.7764, 28.5329)
  line L514 (8.7764, 28.5329) -> (8.788, 28.5496)
  line L515 (8.788, 28.5496) -> (8.8018, 28.5661)
  line L516 (8.8018, 28.5661) -> (8.8176, 28.5825)
  line L517 (8.8176, 28.5825) -> (8.8355, 28.5985)
  line L518 (8.8355, 28.5985) -> (8.8556, 28.6144)
  line L519 (8.8556, 28.6144) -> (8.8777, 28.6299)
  line L520 (8.9019, 28.6451) -> (8.9282, 28.66)
  line L521 (8.8777, 28.6299) -> (8.9019, 28.6451)
  line L522 (8.8777, 31.0603) -> (8.9019, 31.0451)
  line L523 (8.8176, 31.1078) -> (8.8355, 31.0917)
  line L524 (8.8355, 31.0917) -> (8.8556, 31.0759)
  line L525 (8.8556, 31.0759) -> (8.8777, 31.0603)
  line L526 (8.9019, 31.0451) -> (8.9282, 31.0302)
  line L527 (8.8018, 31.1241) -> (8.8176, 31.1078)
  line L528 (8.788, 31.1407) -> (8.8018, 31.1241)
  line L529 (8.7764, 31.1574) -> (8.788, 31.1407)
  line L530 (8.7669, 31.1742) -> (8.7764, 31.1574)
  line L531 (8.7595, 31.1912) -> (8.7669, 31.1742)
  line L532 (8.7542, 31.2082) -> (8.7595, 31.1912)
  line L533 (8.7511, 31.2253) -> (8.7542, 31.2082)
  line L534 (8.75, 31.2424) -> (8.7511, 31.2253)
  line L535 (8.75, 31.4159) -> (8.75, 31.2424)
  line L536 (8.75, 31.4159) -> (8.75, 31.5894)
  line L537 (8.75, 31.5894) -> (8.7511, 31.6065)
  line L538 (8.7511, 31.6065) -> (8.7542, 31.6236)
  line L539 (8.7542, 31.6236) -> (8.7595, 31.6407)
  line L540 (8.9871, 25.547) -> (9.0196, 25.5607)
  line L541 (9.0196, 25.5607) -> (9.0542, 25.5739)
  line L542 (8.7511, 25.3234) -> (8.7542, 25.3405)
  line L543 (8.7542, 25.3405) -> (8.7595, 25.3575)
  line L544 (8.7595, 25.3575) -> (8.7669, 25.3745)
  line L545 (8.7669, 25.3745) -> (8.7764, 25.3913)
  line L546 (8.7764, 25.3913) -> (8.788, 25.408)
  line L547 (8.788, 25.408) -> (8.8018, 25.4245)
  line L548 (8.8018, 25.4245) -> (8.8176, 25.4409)
  line L549 (8.8176, 25.4409) -> (8.8355, 25.457)
  line L550 (8.8355, 25.457) -> (8.8556, 25.4728)
  line L551 (8.8556, 25.4728) -> (8.8777, 25.4883)
  line L552 (8.9019, 25.5035) -> (8.9282, 25.5184)
  line L553 (8.9282, 25.5184) -> (8.9566, 25.5329)
  line L554 (8.9566, 25.5329) -> (8.9871, 25.547)
  line L555 (8.8777, 25.4883) -> (8.9019, 25.5035)
  line L556 (8.7595, 31.6407) -> (8.7669, 31.6577)
  line L557 (8.7764, 31.6745) -> (8.788, 31.6912)
  line L558 (8.788, 31.6912) -> (8.8018, 31.7077)
  line L559 (8.8018, 31.7077) -> (8.8176, 31.724)
  line L560 (8.8176, 31.724) -> (8.8355, 31.7401)
  line L561 (8.8355, 31.7401) -> (8.8556, 31.756)
  line L562 (8.8556, 31.756) -> (8.8777, 31.7715)
  line L563 (8.7669, 31.6577) -> (8.7764, 31.6745)
  line L564 (8.75, 37.6991) -> (8.75, 37.5256)
  line L565 (8.75, 37.5256) -> (8.7511, 37.5085)
  line L566 (8.7511, 37.5085) -> (8.7542, 37.4914)
  line L567 (8.7542, 37.4914) -> (8.7595, 37.4743)
  line L568 (8.7595, 37.4743) -> (8.7669, 37.4574)
  line L569 (8.7669, 37.4574) -> (8.7764, 37.4405)
  line L570 (8.7764, 37.4405) -> (8.788, 37.4238)
  line L571 (8.788, 37.4238) -> (8.8018, 37.4073)
  line L572 (8.8018, 37.4073) -> (8.8176, 37.391)
  line L573 (8.8176, 37.391) -> (8.8355, 37.3749)
  line L574 (8.8355, 37.3749) -> (8.8556, 37.3591)
  line L575 (8.7511, 34.7481) -> (8.7542, 34.7652)
  line L576 (8.75, 34.731) -> (8.7511, 34.7481)
  line L577 (8.75, 34.5575) -> (8.75, 34.731)
  line L578 (8.75, 34.5575) -> (8.75, 34.384)
  line L579 (8.75, 34.384) -> (8.7511, 34.3669)
  line L580 (8.7511, 34.3669) -> (8.7542, 34.3498)
  line L581 (8.7542, 34.3498) -> (8.7595, 34.3327)
  line L582 (8.7595, 34.3327) -> (8.7669, 34.3158)
  line L583 (8.7669, 34.3158) -> (8.7764, 34.2989)
  line L584 (8.7764, 34.2989) -> (8.788, 34.2822)
  line L585 (8.788, 34.2822) -> (8.8018, 34.2657)
  line L586 (8.8018, 34.2657) -> (8.8176, 34.2494)
  line L587 (8.8176, 34.2494) -> (8.8355, 34.2333)
  line L588 (8.8355, 34.2333) -> (8.8556, 34.2175)
  line L589 (8.8556, 34.2175) -> (8.8777, 34.2019)
  line L590 (8.7542, 34.7652) -> (8.7595, 34.7823)
  line L591 (8.7595, 34.7823) -> (8.7669, 34.7992)
  line L592 (9.0196, 34.9855) -> (9.0542, 34.9987)
  line L593 (8.9871, 34.9718) -> (9.0196, 34.9855)
  line L594 (8.9566, 34.9577) -> (8.9871, 34.9718)
  line L595 (8.9282, 34.9432) -> (8.9566, 34.9577)
  line L596 (8.9019, 34.9283) -> (8.9282, 34.9432)
  line L597 (8.8777, 34.9131) -> (8.9019, 34.9283)
  line L598 (8.8556, 34.8976) -> (8.8777, 34.9131)
  line L599 (8.7764, 34.8161) -> (8.788, 34.8328)
  line L600 (8.788, 34.8328) -> (8.8018, 34.8493)
  line L601 (8.8018, 34.8493) -> (8.8176, 34.8656)
  line L602 (8.8176, 34.8656) -> (8.8355, 34.8817)
  line L603 (8.8355, 34.8817) -> (8.8556, 34.8976)
  line L604 (8.7669, 34.7992) -> (8.7764, 34.8161)
  line L605 (9.0542, 34.1164) -> (11, 33.4082)
  line L606 (8.8777, 31.7715) -> (8.9019, 31.7867)
  line L607 (8.9019, 31.7867) -> (8.9282, 31.8016)
  line L608 (8.9282, 31.8016) -> (8.9566, 31.8161)
  line L609 (8.9566, 31.8161) -> (8.9871, 31.8302)
  line L610 (8.9871, 31.8302) -> (9.0196, 31.8439)
  line L611 (9.0196, 31.8439) -> (9.0542, 31.8571)
  line L612 (9.0542, 31.8571) -> (11, 32.5653)
  line L613 (11, 33.4082) -> (11, 32.9867)
  line L614 (11, 32.5653) -> (11, 32.9867)
  line L615 (8.8777, 34.2019) -> (8.9019, 34.1867)
  line L616 (8.9019, 34.1867) -> (8.9282, 34.1718)
  line L617 (8.9282, 34.1718) -> (8.9566, 34.1573)
  line L618 (8.9566, 34.1573) -> (8.9871, 34.1432)
  line L619 (9.0196, 34.1296) -> (9.0542, 34.1164)
  line L620 (8.9871, 34.1432) -> (9.0196, 34.1296)
  line L621 (8.9282, 28.66) -> (8.9566, 28.6745)
  line L622 (8.9566, 28.6745) -> (8.9871, 28.6886)
  line L623 (8.9871, 28.6886) -> (9.0196, 28.7023)
  line L624 (9.0542, 28.7155) -> (11, 29.4237)
  line L625 (8.9282, 31.0302) -> (8.9566, 31.0157)
  line L626 (8.9566, 31.0157) -> (8.9871, 31.0016)
  line L627 (8.9871, 31.0016) -> (9.0196, 30.988)
  line L628 (9.0196, 30.988) -> (9.0542, 30.9748)
  line L629 (11, 29.4237) -> (11, 29.8451)
  line L630 (11, 30.2666) -> (11, 29.8451)
  line L631 (9.0542, 30.9748) -> (11, 30.2666)
  line L632 (9.0196, 28.7023) -> (9.0542, 28.7155)
  line L633 (8.9566, 37.2989) -> (8.9871, 37.2848)
  line L634 (8.9871, 37.2848) -> (9.0196, 37.2712)
  line L635 (9.0196, 37.2712) -> (9.0542, 37.258)
  line L636 (9.0542, 34.9987) -> (11, 35.7069)
  line L637 (9.0542, 37.258) -> (11, 36.5497)
  line L638 (8.8777, 37.3435) -> (8.9019, 37.3283)
  line L639 (8.9019, 37.3283) -> (8.9282, 37.3134)
  line L640 (8.9282, 37.3134) -> (8.9566, 37.2989)
  line L641 (11, 36.5497) -> (11, 36.1283)
  line L642 (11, 35.7069) -> (11, 36.1283)
  line L643 (8.8556, 37.3591) -> (8.8777, 37.3435)
  line L644 (9.0196, 88.3925) -> (9.0542, 88.4058)
  line L645 (9.0542, 88.4058) -> (11, 89.114)
  line L646 (11, 89.114) -> (11, 89.5354)
  line L647 (11, 89.9568) -> (11, 89.5354)
  line L648 (9.0542, 90.665) -> (11, 89.9568)
  line L649 (9.0196, 90.6782) -> (9.0542, 90.665)
  line L650 (8.8556, 90.7661) -> (8.8777, 90.7506)
  line L651 (8.8777, 90.7506) -> (8.9019, 90.7354)
  line L652 (8.9019, 90.7354) -> (8.9282, 90.7205)
  line L653 (8.9282, 90.7205) -> (8.9566, 90.706)
  line L654 (8.9566, 90.706) -> (8.9871, 90.6919)
  line L655 (8.9871, 90.6919) -> (9.0196, 90.6782)
  line L656 (8.8355, 90.782) -> (8.8556, 90.7661)
  line L657 (8.8176, 90.7981) -> (8.8355, 90.782)
  line L658 (8.8018, 90.8144) -> (8.8176, 90.7981)
  line L659 (8.788, 90.8309) -> (8.8018, 90.8144)
  line L660 (8.7764, 90.8476) -> (8.788, 90.8309)
  line L661 (8.7669, 90.8645) -> (8.7764, 90.8476)
  line L662 (8.7595, 90.8814) -> (8.7669, 90.8645)
  line L663 (8.7542, 90.8985) -> (8.7595, 90.8814)
  line L664 (8.7511, 90.9156) -> (8.7542, 90.8985)
  line L665 (8.75, 90.9327) -> (8.7511, 90.9156)
  line L666 (8.8018, 91.398) -> (8.8176, 91.4143)
  line L667 (8.8176, 91.4143) -> (8.8355, 91.4304)
  line L668 (8.8355, 91.4304) -> (8.8556, 91.4462)
  line L669 (8.8556, 91.4462) -> (8.8777, 91.4618)
  line L670 (8.8777, 91.4618) -> (8.9019, 91.477)
  line L671 (8.9019, 91.477) -> (8.9282, 91.4919)
  line L672 (8.9282, 91.4919) -> (8.9566, 91.5064)
  line L673 (8.9566, 91.5064) -> (8.9871, 91.5205)
  line L674 (8.9871, 91.5205) -> (9.0196, 91.5341)
  line L675 (9.0196, 91.5341) -> (9.0542, 91.5473)
  line L676 (9.0542, 91.5473) -> (11, 92.2556)
  line L677 (11, 92.2556) -> (11, 92.677)
  line L678 (11, 93.0984) -> (11, 92.677)
  line L679 (9.0542, 93.8066) -> (11, 93.0984)
  line L680 (8.788, 91.3815) -> (8.8018, 91.398)
  line L681 (8.8777, 93.8922) -> (8.9019, 93.877)
  line L682 (8.8176, 93.9397) -> (8.8355, 93.9236)
  line L683 (8.8556, 93.9077) -> (8.8777, 93.8922)
  line L684 (8.9019, 93.877) -> (8.9282, 93.8621)
  line L685 (8.9282, 93.8621) -> (8.9566, 93.8476)
  line L686 (8.9566, 93.8476) -> (8.9871, 93.8335)
  line L687 (8.9871, 93.8335) -> (9.0196, 93.8198)
  line L688 (9.0196, 93.8198) -> (9.0542, 93.8066)
  line L689 (8.8355, 93.9236) -> (8.8556, 93.9077)
  line L690 (8.75, 94.2478) -> (7.8414, 94.2478)
  line L691 (8.75, 94.2478) -> (8.75, 94.0743)
  line L692 (8.75, 94.0743) -> (8.7511, 94.0572)
  line L693 (8.7511, 94.0572) -> (8.7542, 94.0401)
  line L694 (8.7595, 94.023) -> (8.7669, 94.0061)
  line L695 (8.7669, 94.0061) -> (8.7764, 93.9892)
  line L696 (8.7764, 93.9892) -> (8.788, 93.9725)
  line L697 (8.788, 93.9725) -> (8.8018, 93.956)
  line L698 (8.8018, 93.956) -> (8.8176, 93.9397)
  line L699 (8.7542, 94.0401) -> (8.7595, 94.023)
  line L700 (8.8777, 94.6034) -> (8.9019, 94.6186)
  line L701 (8.9019, 94.6186) -> (8.9282, 94.6335)
  line L702 (8.9282, 94.6335) -> (8.9566, 94.648)
  line L703 (8.75, 94.2478) -> (8.75, 94.4213)
  line L704 (8.75, 94.4213) -> (8.7511, 94.4384)
  line L705 (8.7511, 94.4384) -> (8.7542, 94.4555)
  line L706 (8.7542, 94.4555) -> (8.7595, 94.4725)
  line L707 (8.8556, 94.5878) -> (8.8777, 94.6034)
  line L708 (8.7595, 94.4725) -> (8.7669, 94.4895)
  line L709 (8.7669, 94.4895) -> (8.7764, 94.5064)
  line L710 (8.7764, 94.5064) -> (8.788, 94.5231)
  line L711 (8.788, 94.5231) -> (8.8018, 94.5396)
  line L712 (8.8176, 94.5559) -> (8.8355, 94.572)
  line L713 (8.8355, 94.572) -> (8.8556, 94.5878)
  line L714 (8.8018, 94.5396) -> (8.8176, 94.5559)
  line L715 (8.9566, 94.648) -> (8.9871, 94.6621)
  line L716 (8.9871, 94.6621) -> (9.0196, 94.6757)
  line L717 (9.0196, 94.6757) -> (9.0542, 94.6889)
  line L718 (9.0542, 94.6889) -> (11, 95.3971)
  line L719 (11, 95.3971) -> (11, 95.8186)
  line L720 (9.0542, 96.9482) -> (11, 96.24)
  line L721 (8.9871, 96.9751) -> (9.0196, 96.9614)
  line L722 (8.9566, 96.9892) -> (8.9871, 96.9751)
  line L723 (9.0196, 96.9614) -> (9.0542, 96.9482)
  line L724 (11, 96.24) -> (11, 95.8186)
  line L725 (8.9282, 97.0037) -> (8.9566, 96.9892)
  line L726 (8.7669, 97.1476) -> (8.7764, 97.1308)
  line L727 (8.7764, 97.1308) -> (8.788, 97.1141)
  line L728 (8.788, 97.1141) -> (8.8018, 97.0976)
  line L729 (8.8018, 97.0976) -> (8.8176, 97.0813)
  line L730 (8.8176, 97.0813) -> (8.8355, 97.0652)
  line L731 (8.8355, 97.0652) -> (8.8556, 97.0493)
  line L732 (8.8556, 97.0493) -> (8.8777, 97.0338)
  line L733 (8.8777, 97.0338) -> (8.9019, 97.0186)
  line L734 (8.9019, 97.0186) -> (8.9282, 97.0037)
  line L735 (8.788, 97.6646) -> (8.8018, 97.6812)
  line L736 (8.8018, 97.6812) -> (8.8176, 97.6975)
  line L737 (8.8176, 97.6975) -> (8.8355, 97.7136)
  line L738 (8.8355, 97.7136) -> (8.8556, 97.7294)
  line L739 (8.8556, 97.7294) -> (8.8777, 97.745)
  line L740 (8.7669, 97.6311) -> (8.7764, 97.6479)
  line L741 (8.7764, 97.6479) -> (8.788, 97.6646)
  line L742 (8.8777, 97.745) -> (8.9019, 97.7602)
  line L743 (8.9019, 97.7602) -> (8.9282, 97.7751)
  line L744 (8.9282, 97.7751) -> (8.9566, 97.7896)
  line L745 (8.9566, 97.7896) -> (8.9871, 97.8037)
  line L746 (8.9871, 97.8037) -> (9.0196, 97.8173)
  line L747 (8.75, 97.3894) -> (8.75, 97.5629)
  line L748 (8.75, 97.5629) -> (8.7511, 97.58)
  line L749 (8.7511, 97.58) -> (8.7542, 97.5971)
  line L750 (8.7595, 97.1646) -> (8.7669, 97.1476)
  line L751 (8.7542, 97.1816) -> (8.7595, 97.1646)
  line L752 (8.7511, 97.1988) -> (8.7542, 97.1816)
  line L753 (8.75, 97.2159) -> (8.7511, 97.1988)
  line L754 (8.75, 97.3894) -> (8.75, 97.2159)
  line L755 (8.7542, 97.5971) -> (8.7595, 97.6141)
  line L756 (8.7595, 97.6141) -> (8.7669, 97.6311)
  line L757 (11, 98.5387) -> (11, 98.9602)
  line L758 (9.0196, 97.8173) -> (9.0542, 97.8305)
  line L759 (9.0542, 97.8305) -> (11, 98.5387)
  line L760 (11, 99.3816) -> (11, 98.9602)
  line L761 (9.0542, 100.0898) -> (11, 99.3816)
  line L762 (8.9282, 100.1453) -> (8.9566, 100.1308)
  line L763 (8.9566, 100.1308) -> (8.9871, 100.1167)
  line L764 (8.9871, 100.1167) -> (9.0196, 100.103)
  line L765 (9.0196, 100.103) -> (9.0542, 100.0898)
  line L766 (8.7669, 100.2892) -> (8.7764, 100.2724)
  line L767 (8.75, 100.531) -> (8.75, 100.3575)
  line L768 (8.75, 100.3575) -> (8.7511, 100.3403)
  line L769 (8.9019, 100.1602) -> (8.9282, 100.1453)
  line L770 (8.8777, 100.1754) -> (8.9019, 100.1602)
  line L771 (8.8556, 100.1909) -> (8.8777, 100.1754)
  line L772 (8.8355, 100.2068) -> (8.8556, 100.1909)
  line L773 (8.8176, 100.2228) -> (8.8355, 100.2068)
  line L774 (8.8018, 100.2392) -> (8.8176, 100.2228)
  line L775 (8.7764, 100.2724) -> (8.788, 100.2557)
  line L776 (8.788, 100.2557) -> (8.8018, 100.2392)
  line L777 (8.7595, 100.3062) -> (8.7669, 100.2892)
  line L778 (8.7542, 100.3232) -> (8.7595, 100.3062)
  line L779 (8.7511, 100.3403) -> (8.7542, 100.3232)
  line L780 (8.75, 91.1062) -> (8.75, 91.2797)
  line L781 (8.75, 91.2797) -> (8.7511, 91.2968)
  line L782 (8.7511, 91.2968) -> (8.7542, 91.3139)
  line L783 (8.7542, 91.3139) -> (8.7595, 91.331)
  line L784 (8.7595, 91.331) -> (8.7669, 91.3479)
  line L785 (8.7669, 91.3479) -> (8.7764, 91.3648)
  line L786 (8.7764, 91.3648) -> (8.788, 91.3815)
  line L787 (8.75, 91.1062) -> (8.75, 90.9327)
  line L788 (8.8176, 75.0901) -> (8.8355, 75.074)
  line L789 (8.8355, 75.074) -> (8.8556, 75.0582)
  line L790 (8.8556, 75.0582) -> (8.8777, 75.0426)
  line L791 (8.8777, 75.0426) -> (8.9019, 75.0274)
  line L792 (8.9019, 75.0274) -> (8.9282, 75.0125)
  line L793 (8.9566, 74.998) -> (8.9871, 74.9839)
  line L794 (8.9871, 74.9839) -> (9.0196, 74.9703)
  line L795 (9.0196, 74.9703) -> (9.0542, 74.9571)
  line L796 (8.9282, 75.0125) -> (8.9566, 74.998)
  line L797 (8.75, 75.3982) -> (7.9383, 75.3982)
  line L798 (8.75, 75.2247) -> (8.7511, 75.2076)
  line L799 (8.8018, 75.1064) -> (8.8176, 75.0901)
  line L800 (8.788, 75.123) -> (8.8018, 75.1064)
  line L801 (8.7764, 75.1397) -> (8.788, 75.123)
  line L802 (8.7669, 75.1565) -> (8.7764, 75.1397)
  line L803 (8.7595, 75.1735) -> (8.7669, 75.1565)
  line L804 (8.7542, 75.1905) -> (8.7595, 75.1735)
  line L805 (8.7511, 75.2076) -> (8.7542, 75.1905)
  line L806 (8.75, 75.3982) -> (8.75, 75.2247)
  line L807 (8.75, 75.3982) -> (8.75, 75.5717)
  line L808 (8.75, 75.5717) -> (8.7511, 75.5888)
  line L809 (8.7511, 75.5888) -> (8.7542, 75.6059)
  line L810 (8.7542, 75.6059) -> (8.7595, 75.623)
  line L811 (8.8176, 75.7063) -> (8.8355, 75.7224)
  line L812 (8.8355, 75.7224) -> (8.8556, 75.7383)
  line L813 (8.7595, 75.623) -> (8.7669, 75.64)
  line L814 (8.7669, 75.64) -> (8.7764, 75.6568)
  line L815 (8.7764, 75.6568) -> (8.788, 75.6735)
  line L816 (8.8018, 75.69) -> (8.8176, 75.7063)
  line L817 (8.8556, 75.7383) -> (8.8777, 75.7538)
  line L818 (8.8777, 75.7538) -> (8.9019, 75.769)
  line L819 (8.9019, 75.769) -> (8.9282, 75.7839)
  line L820 (8.9282, 75.7839) -> (8.9566, 75.7984)
  line L821 (8.9566, 75.7984) -> (8.9871, 75.8125)
  line L822 (8.788, 75.6735) -> (8.8018, 75.69)
  line L823 (9.0542, 74.9571) -> (11, 74.2489)
  line L824 (11, 74.2489) -> (11, 73.8274)
  line L825 (11, 73.406) -> (11, 73.8274)
  line L826 (9.0542, 72.6978) -> (11, 73.406)
  line L827 (9.0196, 72.6846) -> (9.0542, 72.6978)
  line L828 (8.9871, 72.6709) -> (9.0196, 72.6846)
  line L829 (8.7764, 72.5152) -> (8.788, 72.5319)
  line L830 (8.788, 72.5319) -> (8.8018, 72.5484)
  line L831 (8.8018, 72.5484) -> (8.8176, 72.5648)
  line L832 (8.8176, 72.5648) -> (8.8355, 72.5808)
  line L833 (8.8355, 72.5808) -> (8.8556, 72.5967)
  line L834 (8.8556, 72.5967) -> (8.8777, 72.6122)
  line L835 (8.8777, 72.6122) -> (8.9019, 72.6274)
  line L836 (8.9019, 72.6274) -> (8.9282, 72.6423)
  line L837 (8.9282, 72.6423) -> (8.9566, 72.6568)
  line L838 (8.9566, 72.6568) -> (8.9871, 72.6709)
  line L839 (8.7669, 72.4984) -> (8.7764, 72.5152)
  line L840 (8.7595, 72.4814) -> (8.7669, 72.4984)
  line L841 (8.7542, 72.4644) -> (8.7595, 72.4814)
  line L842 (8.7511, 72.4472) -> (8.7542, 72.4644)
  line L843 (8.75, 72.4301) -> (8.7511, 72.4472)
  line L844 (8.75, 72.2566) -> (8.75, 72.4301)
  line L845 (8.75, 72.2566) -> (8.75, 72.0831)
  line L846 (8.75, 72.0831) -> (8.7511, 72.066)
  line L847 (8.7511, 72.066) -> (8.7542, 72.0489)
  line L848 (8.7542, 72.0489) -> (8.7595, 72.0319)
  line L849 (8.7595, 72.0319) -> (8.7669, 72.0149)
  line L850 (8.7669, 72.0149) -> (8.7764, 71.9981)
  line L851 (8.7764, 71.9981) -> (8.788, 71.9814)
  line L852 (8.788, 71.9814) -> (8.8018, 71.9648)
  line L853 (8.8018, 71.9648) -> (8.8176, 71.9485)
  line L854 (8.8176, 71.9485) -> (8.8355, 71.9324)
  line L855 (8.8355, 71.9324) -> (8.8556, 71.9166)
  line L856 (8.8556, 71.9166) -> (8.8777, 71.901)
  line L857 (8.8777, 71.901) -> (8.9019, 71.8858)
  line L858 (8.9019, 71.8858) -> (8.9282, 71.8709)
  line L859 (8.9282, 71.8709) -> (8.9566, 71.8564)
  line L860 (8.9566, 71.8564) -> (8.9871, 71.8423)
  line L861 (9.0196, 71.8287) -> (9.0542, 71.8155)
  line L862 (9.0542, 71.8155) -> (11, 71.1073)
  line L863 (11, 71.1073) -> (11, 70.6858)
  line L864 (11, 70.2644) -> (11, 70.6858)
  line L865 (9.0542, 69.5562) -> (11, 70.2644)
  line L866 (8.9871, 71.8423) -> (9.0196, 71.8287)
  line L867 (8.8176, 69.4232) -> (8.8355, 69.4392)
  line L868 (8.8018, 69.4068) -> (8.8176, 69.4232)
  line L869 (8.788, 69.3903) -> (8.8018, 69.4068)
  line L870 (8.7764, 69.3736) -> (8.788, 69.3903)
  line L871 (8.7669, 69.3568) -> (8.7764, 69.3736)
  line L872 (8.7595, 69.3398) -> (8.7669, 69.3568)
  line L873 (8.7542, 69.3228) -> (8.7595, 69.3398)
  line L874 (8.7511, 69.3057) -> (8.7542, 69.3228)
  line L875 (8.75, 69.2885) -> (8.7511, 69.3057)
  line L876 (8.75, 69.115) -> (8.75, 69.2885)
  line L877 (8.75, 69.115) -> (8.75, 68.9416)
  line L878 (8.75, 68.9416) -> (8.7511, 68.9244)
  line L879 (8.7542, 68.9073) -> (8.7595, 68.8903)
  line L880 (8.7595, 68.8903) -> (8.7669, 68.8733)
  line L881 (8.7669, 68.8733) -> (8.7764, 68.8565)
  line L882 (8.7511, 68.9244) -> (8.7542, 68.9073)
  line L883 (8.7764, 68.8565) -> (8.788, 68.8398)
  line L884 (8.788, 68.8398) -> (8.8018, 68.8232)
  line L885 (8.8018, 68.8232) -> (8.8176, 68.8069)
  line L886 (8.8176, 68.8069) -> (8.8355, 68.7908)
  line L887 (8.8355, 68.7908) -> (8.8556, 68.775)
  line L888 (8.8556, 68.775) -> (8.8777, 68.7595)
  line L889 (8.8777, 68.7595) -> (8.9019, 68.7442)
  line L890 (8.9019, 68.7442) -> (8.9282, 68.7294)
  line L891 (8.9282, 68.7294) -> (8.9566, 68.7149)
  line L892 (8.9566, 68.7149) -> (8.9871, 68.7008)
  line L893 (8.9871, 68.7008) -> (9.0196, 68.6871)
  line L894 (9.0196, 68.6871) -> (9.0542, 68.6739)
  line L895 (9.0542, 68.6739) -> (11, 67.9657)
  line L896 (11, 67.9657) -> (11, 67.5442)
  line L897 (11, 67.1228) -> (11, 67.5442)
  line L898 (9.0542, 66.4146) -> (11, 67.1228)
  line L899 (8.8777, 66.329) -> (8.9019, 66.3443)
  line L900 (8.9019, 66.3443) -> (8.9282, 66.3591)
  line L901 (8.9282, 66.3591) -> (8.9566, 66.3736)
  line L902 (8.9566, 66.3736) -> (8.9871, 66.3877)
  line L903 (9.0196, 66.4014) -> (9.0542, 66.4146)
  line L904 (8.9871, 66.3877) -> (9.0196, 66.4014)
  line L905 (8.75, 65.9734) -> (8.75, 66.1469)
  line L906 (8.75, 66.1469) -> (8.7511, 66.1641)
  line L907 (8.8556, 66.3135) -> (8.8777, 66.329)
  line L908 (8.8355, 66.2977) -> (8.8556, 66.3135)
  line L909 (8.8176, 66.2816) -> (8.8355, 66.2977)
  line L910 (8.8018, 66.2652) -> (8.8176, 66.2816)
  line L911 (8.7764, 66.232) -> (8.788, 66.2487)
  line L912 (8.7669, 66.2152) -> (8.7764, 66.232)
  line L913 (8.7595, 66.1982) -> (8.7669, 66.2152)
  line L914 (8.7542, 66.1812) -> (8.7595, 66.1982)
  line L915 (8.7511, 66.1641) -> (8.7542, 66.1812)
  line L916 (8.788, 66.2487) -> (8.8018, 66.2652)
  line L917 (8.7511, 65.7828) -> (8.7542, 65.7657)
  line L918 (8.8018, 65.6816) -> (8.8176, 65.6653)
  line L919 (8.788, 65.6982) -> (8.8018, 65.6816)
  line L920 (8.7764, 65.7149) -> (8.788, 65.6982)
  line L921 (8.7669, 65.7317) -> (8.7764, 65.7149)
  line L922 (8.7595, 65.7487) -> (8.7669, 65.7317)
  line L923 (8.7542, 65.7657) -> (8.7595, 65.7487)
  line L924 (8.75, 65.8) -> (8.7511, 65.7828)
  line L925 (8.75, 65.9734) -> (8.75, 65.8)
  line L926 (8.8176, 65.6653) -> (8.8355, 65.6492)
  line L927 (8.8355, 65.6492) -> (8.8556, 65.6334)
  line L928 (8.8556, 65.6334) -> (8.8777, 65.6179)
  line L929 (8.8777, 65.6179) -> (8.9019, 65.6026)
  line L930 (8.9019, 65.6026) -> (8.9282, 65.5878)
  line L931 (8.9566, 65.5733) -> (8.9871, 65.5592)
  line L932 (8.9871, 65.5592) -> (9.0196, 65.5455)
  line L933 (9.0196, 65.5455) -> (9.0542, 65.5323)
  line L934 (8.9282, 65.5878) -> (8.9566, 65.5733)
  line L935 (11, 64.8241) -> (11, 64.4026)
  line L936 (11, 63.9812) -> (11, 64.4026)
  line L937 (9.0542, 63.273) -> (11, 63.9812)
  line L938 (9.0542, 65.5323) -> (11, 64.8241)
  line L939 (8.8355, 63.1561) -> (8.8556, 63.1719)
  line L940 (8.8556, 63.1719) -> (8.8777, 63.1874)
  line L941 (8.8777, 63.1874) -> (8.9019, 63.2027)
  line L942 (8.9019, 63.2027) -> (8.9282, 63.2175)
  line L943 (8.9282, 63.2175) -> (8.9566, 63.232)
  line L944 (8.9566, 63.232) -> (8.9871, 63.2461)
  line L945 (8.9871, 63.2461) -> (9.0196, 63.2598)
  line L946 (9.0196, 63.2598) -> (9.0542, 63.273)
  line L947 (8.75, 62.8319) -> (8.75, 63.0053)
  line L948 (8.75, 63.0053) -> (8.7511, 63.0225)
  line L949 (8.7511, 63.0225) -> (8.7542, 63.0396)
  line L950 (8.7542, 63.0396) -> (8.7595, 63.0566)
  line L951 (8.7595, 63.0566) -> (8.7669, 63.0736)
  line L952 (8.7669, 63.0736) -> (8.7764, 63.0904)
  line L953 (8.7764, 63.0904) -> (8.788, 63.1071)
  line L954 (8.8018, 63.1237) -> (8.8176, 63.14)
  line L955 (8.8176, 63.14) -> (8.8355, 63.1561)
  line L956 (8.788, 63.1071) -> (8.8018, 63.1237)
  line L957 (8.8355, 69.4392) -> (8.8556, 69.4551)
  line L958 (8.8556, 69.4551) -> (8.8777, 69.4706)
  line L959 (8.8777, 69.4706) -> (8.9019, 69.4858)
  line L960 (8.9019, 69.4858) -> (8.9282, 69.5007)
  line L961 (8.9282, 69.5007) -> (8.9566, 69.5152)
  line L962 (8.9566, 69.5152) -> (8.9871, 69.5293)
  line L963 (8.9871, 69.5293) -> (9.0196, 69.543)
  line L964 (9.0196, 69.543) -> (9.0542, 69.5562)
  line L965 (8.9019, 50.6363) -> (8.9282, 50.6512)
  line L966 (9.0542, 52.9659) -> (11, 52.2577)
  line L967 (11, 52.2577) -> (11, 51.8363)
  line L968 (11, 51.4149) -> (11, 51.8363)
  line L969 (9.0542, 50.7066) -> (11, 51.4149)
  line L970 (9.0196, 50.6934) -> (9.0542, 50.7066)
  line L971 (8.9871, 50.6798) -> (9.0196, 50.6934)
  line L972 (8.9566, 50.6657) -> (8.9871, 50.6798)
  line L973 (8.9282, 50.6512) -> (8.9566, 50.6657)
  line L974 (8.8777, 50.6211) -> (8.9019, 50.6363)
  line L975 (8.788, 53.1318) -> (8.8018, 53.1153)
  line L976 (8.8018, 53.1153) -> (8.8176, 53.099)
  line L977 (8.7764, 53.1485) -> (8.788, 53.1318)
  line L978 (8.7669, 53.1653) -> (8.7764, 53.1485)
  line L979 (8.75, 53.2336) -> (8.7511, 53.2165)
  line L980 (8.7511, 53.2165) -> (8.7542, 53.1994)
  line L981 (8.7542, 53.1994) -> (8.7595, 53.1823)
  line L982 (8.7595, 53.1823) -> (8.7669, 53.1653)
  line L983 (8.75, 53.4071) -> (8.75, 53.2336)
  line L984 (8.75, 53.4071) -> (8.75, 53.5806)
  line L985 (8.75, 53.5806) -> (8.7511, 53.5977)
  line L986 (8.7511, 53.5977) -> (8.7542, 53.6148)
  line L987 (8.7542, 53.6148) -> (8.7595, 53.6318)
  line L988 (8.7595, 53.6318) -> (8.7669, 53.6488)
  line L989 (8.7669, 53.6488) -> (8.7764, 53.6656)
  line L990 (8.7764, 53.6656) -> (8.788, 53.6823)
  line L991 (8.788, 53.6823) -> (8.8018, 53.6989)
  line L992 (8.8018, 53.6989) -> (8.8176, 53.7152)
  line L993 (8.8176, 53.7152) -> (8.8355, 53.7313)
  line L994 (8.8355, 53.7313) -> (8.8556, 53.7471)
  line L995 (8.8556, 53.7471) -> (8.8777, 53.7627)
  line L996 (8.8556, 62.4918) -> (8.8777, 62.4763)
  line L997 (8.8355, 62.5076) -> (8.8556, 62.4918)
  line L998 (8.8176, 62.5237) -> (8.8355, 62.5076)